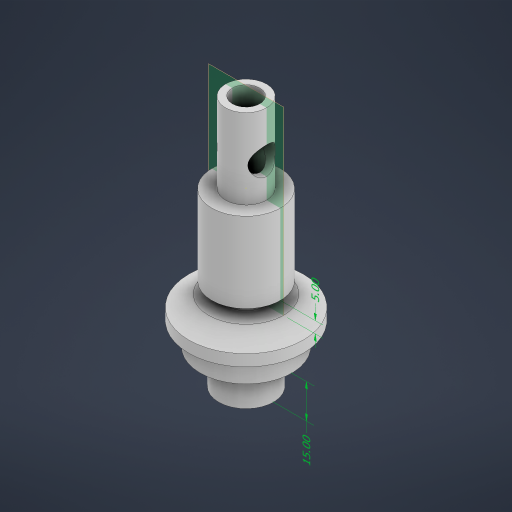
# Autodesk Inventor part: Vtulka
Saved by Autodesk Inventor 2024.3 (Build 283343000, 343)
## iProperties
Created: 2025-07-11
Part Number: Vtulka
Material: Generic
Document SubType Name: Modeling
Designer: LeoFB
Density: 1 g/cm^3
Appearance: Default
Author: LeoFB
Autodesk Inventor part; units mm, degrees
ref_plane "YZ Plane" through (0, 0, 0) normal (1, 0, 0) x (0, 1, 0)
ref_plane "XZ Plane" through (0, 0, 0) normal (0, 1, 0) x (-1, 0, 0)
ref_plane "XY Plane" through (0, 0, 0) normal (0, 0, 1) x (1, 0, 0)
sketch "Sketch2" plane through (0, 0, 0) normal (0, 1, 0) x (-1, 0, 0)
  circle A0 centre (0, 0) radius 9
  dimension "d0" = 18
  constraints: 1 centre point, 1 coincident
  measures "d0" diameter of A0
extrude "Extrusion1" add sketch "Sketch2" along normal blind 35
sketch "Sketch3" plane through (0, 0, 0) normal (0, -1, 0) x (1, 0, 0)
  circle A0 centre (0, 0) radius 15
  dimension "d3" = 30
  constraints: 1 centre point, 1 coincident
  measures "d3" diameter of A0
extrude "Extrusion2" add sketch "Sketch3" along normal blind 35
sketch "Sketch4" plane through (0, -35, 0) normal (0, -1, 0) x (1, 0, 0)
  circle A0 centre (0, 0) radius 9 projected
  circle A1 centre (0, 0) radius 9
  constraints: 1 centre point, 1 coincident
extrude "Extrusion3" add sketch "Sketch4" along normal blind 5
ref_plane "Work Plane1" through (0, -40, 0) normal (0, 0, -1) x (-1, 0, 0)
sketch "Sketch7" plane through (0, -40, 0) normal (0, 0, -1) x (-1, 0, 0)
  point P0 (0, 40)
sketch "Sketch8" plane through (0, -40, 0) normal (0, 0, -1) x (-1, 0, 0)
  line L0 (-9, 0) -> (9, 0) projected
  line L1 (-15, 5) -> (15, 5) projected
  line L2 (0, 0) -> (15, 0) construction
  line L3 (-16.3397, 0) -> (-25, -5)
  line L4 (0, 0) -> (0, -5)
  line L5 (0, -5) -> (-25, -5)
  line L6 (0, 0) -> (-16.3397, 0)
  point P0 (0, 40)
  dimension "d21" = 5
  dimension "d22" = 25
  constraints: 10 end point, 2 perpendicular, 1 collinear, 1 horizontal, 1 midpoint
  measures "d21" distance of L2.start L4.end
  measures "d22" distance of L4.end L5.end
revolve "Revolution1" add sketch "Sketch8" angle 360 about axis through (0, -40, 0) along (0, -1, 0)
sketch "Sketch9" plane through (0, -45, 0) normal (0, -1, 0) x (1, 0, 0)
  circle A0 centre (0, 0) radius 25
  constraints: 1 centre point, 1 coincident
extrude "Extrusion5" add sketch "Sketch9" along normal blind 5
sketch "Sketch10" plane through (0, -50, 0) normal (0, -1, 0) x (1, 0, 0)
  circle A0 centre (0, 0) radius 20
  dimension "d26" = 40
  constraints: 1 centre point, 1 coincident
  measures "d26" diameter of A0
extrude "Extrusion6" add sketch "Sketch10" along normal blind 10
sketch "Sketch11" plane through (0, -60, 0) normal (0, -1, 0) x (1, 0, 0)
  circle A0 centre (0, 0) radius 9 projected
  circle A1 centre (0, 0) radius 12
  dimension "d29" = 24
  constraints: 1 centre point, 1 coincident
  measures "d29" diameter of A1
extrude "Extrusion7" add sketch "Sketch11" along normal blind 15 contours A0 | A1
sketch "Sketch12" plane through (0, 35, 0) normal (0, 1, 0) x (1, 0, 0)
  circle A0 centre (0, 0) radius 6
  dimension "d32" = 12
  constraints: 1 centre point, 1 coincident
  measures "d32" diameter of A0
extrude "Extrusion8" cut sketch "Sketch12" against normal blind 120
sketch "Sketch13" plane through (0, -40, 0) normal (0, 0, -1) x (-1, 0, 0)
  circle A0 centre (0, 55) radius 6
  line L0 (9, 75) -> (-9, 75) projected
  line L1 (9, 40) -> (-9, 40) projected
  point P0 (0, 40)
  dimension "d45" = 12
  dimension "d47" = 15
  constraints: 1 centre point
  measures "d45" diameter of A0
  measures "d47" distance from line of L1 A0.centre
extrude "Extrusion9" cut sketch "Sketch13" along normal mid plane 18
move or copy body "Move Body2" bodies to move or copy 1 copy no rotation origin (0, 0, 0) rotation axis (0, 1, 0) rotation angle -90
body "Solid1"
